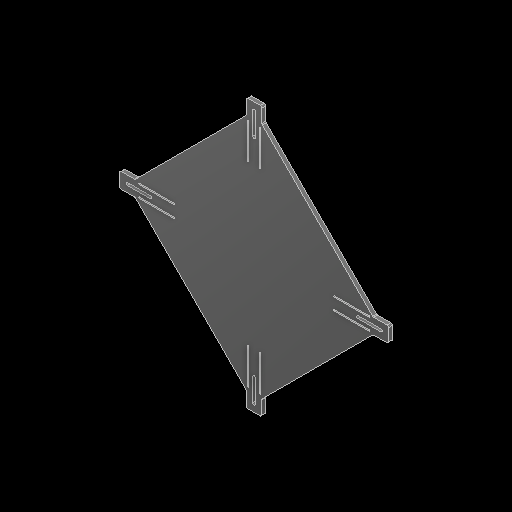
# Autodesk Inventor part: base_plate
Saved by Autodesk Inventor 2026.1 (Build 301233000, 233)
## iProperties
Created: 2025-09-14
Part Number: base_plate
Material: Aluminum 6061
Document SubType Name: Modeling
Designer: drago
Density: 2.7 g/cm^3
Appearance: Smooth - Black
Author: drago
Autodesk Inventor part; units mm, degrees
ref_plane "YZ Plane" through (0, 0, 0) normal (1, 0, 0) x (0, 1, 0)
ref_plane "XZ Plane" through (0, 0, 0) normal (0, 1, 0) x (-1, 0, 0)
ref_plane "XY Plane" through (0, 0, 0) normal (0, 0, 1) x (1, 0, 0)
sketch "Sketch2" plane through (0, 0, 0) normal (0, 0, 1) x (1, 0, 0)
  circle A0 centre (0, 0) radius 327.5 construction
  line L0 (260.6, -21.1) -> (302.8, -21.1) construction
  line L1 (302.8, -21.1) -> (302.8, 21.1) construction
  line L2 (302.8, 21.1) -> (260.6, 21.1) construction
  line L3 (260.6, 21.1) -> (260.6, -21.1) construction
  line L4 (260.6, -21.1) -> (302.8, 21.1) construction
  line L5 (302.8, -21.1) -> (260.6, 21.1) construction
  line L6 (297.2, 15.5) -> (207.0955, 15.5) construction
  line L7 (297.2, 17.1) -> (207.0955, 17.1)
  line L8 (207.0955, 13.9) -> (297.2, 13.9)
  arc A1 (297.2, 13.9) -> (297.2, 17.1) centre (297.2, 15.5) ccw
  arc A2 (207.0955, 17.1) -> (207.0955, 13.9) centre (207.0955, 15.5) ccw
  line L9 (297.2, -15.5) -> (207.0955, -15.5) construction
  line L10 (297.2, -13.9) -> (207.0955, -13.9)
  line L11 (207.0955, -17.1) -> (297.2, -17.1)
  arc A3 (297.2, -17.1) -> (297.2, -13.9) centre (297.2, -15.5) ccw
  arc A4 (207.0955, -13.9) -> (207.0955, -17.1) centre (207.0955, -15.5) ccw
  line L12 (327.5, 0) -> (268.3955, 0) construction
  line L13 (327.5, 3.4) -> (268.3955, 3.4)
  line L14 (268.3955, -3.4) -> (327.5, -3.4)
  arc A5 (327.5, -3.4) -> (327.5, 3.4) centre (327.5, 0) ccw
  arc A6 (268.3955, 3.4) -> (268.3955, -3.4) centre (268.3955, 0) ccw
  line L15 (307.5, -20) -> (347.5, -20)
  line L16 (347.5, -20) -> (347.5, 20)
  line L17 (347.5, 20) -> (307.5, 20)
  line L18 (307.5, 20) -> (307.5, -20)
  line L19 (307.5, -20) -> (347.5, 20) construction
  line L20 (347.5, -20) -> (307.5, 20) construction
  circle A7 centre (327.5, 0) radius 3.4
  arc A8 (-3.4, 268.3955) -> (3.4, 268.3955) centre (0, 268.3955) ccw
  line L21 (-13.9, 207.0955) -> (-13.9, 297.2)
  line L22 (-17.1, 297.2) -> (-17.1, 207.0955)
  line L23 (-15.5, 297.2) -> (-15.5, 207.0955) construction
  line L24 (17.1, 207.0955) -> (17.1, 297.2)
  line L25 (15.5, 297.2) -> (15.5, 207.0955) construction
  line L26 (13.9, 297.2) -> (13.9, 207.0955)
  arc A9 (-17.1, 207.0955) -> (-13.9, 207.0955) centre (-15.5, 207.0955) ccw
  arc A10 (13.9, 207.0955) -> (17.1, 207.0955) centre (15.5, 207.0955) ccw
  line L27 (21.1, 302.8) -> (-21.1, 302.8) construction
  arc A11 (-13.9, 297.2) -> (-17.1, 297.2) centre (-15.5, 297.2) ccw
  arc A12 (17.1, 297.2) -> (13.9, 297.2) centre (15.5, 297.2) ccw
  line L28 (0, 327.5) -> (0, 268.3955) construction
  line L29 (-3.4, 327.5) -> (-3.4, 268.3955)
  line L30 (3.4, 268.3955) -> (3.4, 327.5)
  line L31 (21.1, 260.6) -> (21.1, 302.8) construction
  line L32 (21.1, 302.8) -> (-21.1, 260.6) construction
  line L33 (-21.1, 260.6) -> (21.1, 260.6) construction
  line L34 (21.1, 260.6) -> (-21.1, 302.8) construction
  line L35 (-21.1, 302.8) -> (-21.1, 260.6) construction
  line L36 (-20, 307.5) -> (20, 307.5)
  arc A13 (3.4, 327.5) -> (-3.4, 327.5) centre (0, 327.5) ccw
  circle A14 centre (0, 327.5) radius 3.4
  line L37 (20, 307.5) -> (20, 347.5)
  line L38 (-20, 347.5) -> (-20, 307.5)
  line L39 (20, 307.5) -> (-20, 347.5) construction
  line L40 (20, 347.5) -> (-20, 307.5) construction
  line L41 (20, 347.5) -> (-20, 347.5)
  arc A15 (-268.3955, -3.4) -> (-268.3955, 3.4) centre (-268.3955, 0) ccw
  line L42 (-207.0955, -13.9) -> (-297.2, -13.9)
  line L43 (-297.2, -17.1) -> (-207.0955, -17.1)
  line L44 (-297.2, -15.5) -> (-207.0955, -15.5) construction
  line L45 (-207.0955, 17.1) -> (-297.2, 17.1)
  line L46 (-297.2, 15.5) -> (-207.0955, 15.5) construction
  line L47 (-297.2, 13.9) -> (-207.0955, 13.9)
  arc A16 (-207.0955, -17.1) -> (-207.0955, -13.9) centre (-207.0955, -15.5) ccw
  arc A17 (-207.0955, 13.9) -> (-207.0955, 17.1) centre (-207.0955, 15.5) ccw
  line L48 (-302.8, 21.1) -> (-302.8, -21.1) construction
  arc A18 (-297.2, -13.9) -> (-297.2, -17.1) centre (-297.2, -15.5) ccw
  arc A19 (-297.2, 17.1) -> (-297.2, 13.9) centre (-297.2, 15.5) ccw
  line L49 (-327.5, 0) -> (-268.3955, 0) construction
  line L50 (-327.5, -3.4) -> (-268.3955, -3.4)
  line L51 (-268.3955, 3.4) -> (-327.5, 3.4)
  line L52 (-260.6, 21.1) -> (-302.8, 21.1) construction
  line L53 (-302.8, 21.1) -> (-260.6, -21.1) construction
  line L54 (-260.6, -21.1) -> (-260.6, 21.1) construction
  line L55 (-260.6, 21.1) -> (-302.8, -21.1) construction
  line L56 (-302.8, -21.1) -> (-260.6, -21.1) construction
  line L57 (-307.5, -20) -> (-307.5, 20)
  arc A20 (-327.5, 3.4) -> (-327.5, -3.4) centre (-327.5, 0) ccw
  circle A21 centre (-327.5, 0) radius 3.4
  line L58 (-307.5, 20) -> (-347.5, 20)
  line L59 (-347.5, -20) -> (-307.5, -20)
  line L60 (-307.5, 20) -> (-347.5, -20) construction
  line L61 (-347.5, 20) -> (-307.5, -20) construction
  line L62 (-347.5, 20) -> (-347.5, -20)
  arc A22 (3.4, -268.3955) -> (-3.4, -268.3955) centre (0, -268.3955) ccw
  line L63 (13.9, -207.0955) -> (13.9, -297.2)
  line L64 (17.1, -297.2) -> (17.1, -207.0955)
  line L65 (15.5, -297.2) -> (15.5, -207.0955) construction
  line L66 (-17.1, -207.0955) -> (-17.1, -297.2)
  line L67 (-15.5, -297.2) -> (-15.5, -207.0955) construction
  line L68 (-13.9, -297.2) -> (-13.9, -207.0955)
  arc A23 (17.1, -207.0955) -> (13.9, -207.0955) centre (15.5, -207.0955) ccw
  arc A24 (-13.9, -207.0955) -> (-17.1, -207.0955) centre (-15.5, -207.0955) ccw
  line L69 (-21.1, -302.8) -> (21.1, -302.8) construction
  arc A25 (13.9, -297.2) -> (17.1, -297.2) centre (15.5, -297.2) ccw
  arc A26 (-17.1, -297.2) -> (-13.9, -297.2) centre (-15.5, -297.2) ccw
  line L70 (0, -327.5) -> (0, -268.3955) construction
  line L71 (3.4, -327.5) -> (3.4, -268.3955)
  line L72 (-3.4, -268.3955) -> (-3.4, -327.5)
  line L73 (-21.1, -260.6) -> (-21.1, -302.8) construction
  line L74 (-21.1, -302.8) -> (21.1, -260.6) construction
  line L75 (21.1, -260.6) -> (-21.1, -260.6) construction
  line L76 (-21.1, -260.6) -> (21.1, -302.8) construction
  line L77 (21.1, -302.8) -> (21.1, -260.6) construction
  line L78 (20, -307.5) -> (-20, -307.5)
  arc A27 (-3.4, -327.5) -> (3.4, -327.5) centre (0, -327.5) ccw
  circle A28 centre (0, -327.5) radius 3.4
  line L79 (-20, -307.5) -> (-20, -347.5)
  line L80 (20, -347.5) -> (20, -307.5)
  line L81 (-20, -307.5) -> (20, -347.5) construction
  line L82 (-20, -347.5) -> (20, -307.5) construction
  line L83 (-20, -347.5) -> (20, -347.5)
  line L84 (-20, 307.5) -> (-307.5, 20)
  line L85 (-307.5, -20) -> (-20, -307.5)
  line L86 (307.5, -20) -> (20, -307.5)
  line L87 (20, 307.5) -> (307.5, 20)
  point P0 (281.7, 0)
  point P1 (252.1478, 15.5)
  point P2 (252.1478, -15.5)
  point P3 (297.9478, 0)
  point P4 (15.5, 252.1478)
  point P5 (0, 281.7)
  point P6 (-15.5, 252.1478)
  point P7 (0, 297.9478)
  point P8 (-252.1478, 15.5)
  point P9 (-281.7, 0)
  point P10 (-252.1478, -15.5)
  point P11 (-297.9478, 0)
  point P12 (-15.5, -252.1478)
  point P13 (0, -281.7)
  point P14 (15.5, -252.1478)
  point P15 (0, -297.9478)
  dimension "d26" = 655
  dimension "d110" = 42.2
  dimension "d113" = 42.2
  dimension "d114" = 3.2
  dimension "d115" = 90.1045
  dimension "d116" = 5.6
  dimension "d117" = 3.2
  dimension "d118" = 5.6
  dimension "d119" = 90.1045
  dimension "d122" = 59.1045
  dimension "d123" = 6.8
  dimension "d134" = 40
  dimension "d135" = 40
  dimension "d136" = 6.8
  dimension "d137" = 327.5
  dimension "d138" = 4.7
  dimension "d141" = 360
  constraints: 200 end point, 48 point on circle, 29 centre point, 12 tangent, 8 point on line, 7 midpoint, 7 parallel, 5 horizontal, 4 coincident, 4 perpendicular, 2 collinear, 237 other
  measures "d26" diameter of A0
  measures "d110" distance of L2.end L1.end
  measures "d113" distance between parallel lines of L0 L2
  measures "d114" diameter of A2
  measures "d115" distance of L6.start L6.end
  measures "d116" distance between parallel lines of L2 L6
  measures "d117" diameter of A4
  measures "d118" distance between parallel lines of L0 L9
  measures "d119" distance of L9.start L9.end
  measures "d122" distance of L12.start L12.end
  measures "d123" diameter of A6
  measures "d134" distance of L17.end L16.end
  measures "d135" distance of L15.end L16.end
  measures "d136" diameter of A7
  measures "d137" distance of point (0, 0) A7.centre
  measures "d138" distance between parallel lines of L18 L1
extrude "Extrusion9" add sketch "Sketch2" against normal blind 10 contours L13 L18 L17 L16 L15 L14 A5 | L13 A6 L14 L18 L86 L78 L71 A22 L72 L85 L57 L50 A15 L51 L84 L36 L29 A8 L30 L87 | L36 L30 A13 L29 L38 L41 L37 | L80 L83 L79 L78 L72 A27 L71 | L57 L51 A20 L50 L59 L62 L58
fillet "Fillet7" radius 4 16 edges at (20, 347.5, -5) (20, 307.5, -5) (-20, 347.5, -5) (-20, 307.5, -5) (-347.5, 20, -5) (-307.5, 20, -5) (-347.5, -20, -5) (-307.5, -20, -5) (-20, -347.5, -5) (-20, -307.5, -5) (347.5, -20, -5) (20, -347.5, -5) (307.5, 20, -5) (347.5, 20, -5) (20, -307.5, -5) (307.5, -20, -5)
equation "\"d26\" = ring_outer_diam + bar_width"
equation "\"ring_inner_diam\" = 565"
equation "\"bar_width\" = 40"
equation "\"bar_hole_diam\" = 6.8"
equation "\"ring_outer_diam\" = 615"
equation "\"motor_width\" = 42.2"
equation "\"dist_motor_bar\" = 4.7"
equation "\"motor_slot_diam\" = 3.2"
equation "\"motor_hole_edge_dist\" = 5.6"
equation "\"motor_slot_length\" = 90.1045"
equation "\"bar_slot_diam\" = 6.8"
equation "\"bar_slot_length\" = 59.1045"
equation "\"dist_motor_holes\" = 31"
equation "\"diag_dist_bar_holes_old_fridge\" = 536.791"
body "Solid3"
